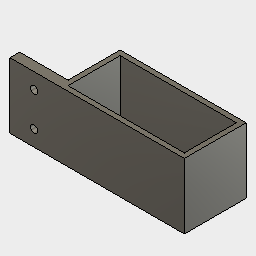
ServoHolder (Autodesk Fusion 360 design; units mm, degrees)
Autodesk Fusion 360 part; units mm, degrees
note: some values were not read from the file. Chosen so that the rebuilt part matches the saved one: which face or edge a step refers to.
sketch "Sketch1" plane through (0, 0, 0) normal (0, 1, 0) x (1, 0, 0)
  line L0 (0, 0) -> (47, 0) construction
  line L1 (47, 0) -> (47, 20.5) construction
  line L2 (47, 20.5) -> (0, 20.5) construction
  line L3 (0, 20.5) -> (0, 0) construction
  line L4 (-0.5, -0.5) -> (47.5, -0.5)
  line L5 (47.5, -0.5) -> (47.5, 21)
  line L6 (47.5, 21) -> (-0.5, 21)
  line L7 (-0.5, 21) -> (-0.5, -0.5)
  dimension "d1" = 47
  dimension "d2" = 20.5
  dimension "d3" = 0.5
  measures "d1" distance of L0.start L0.end
  measures "d2" distance of L0.start L2.end
extrude "Extrude1" add sketch "Sketch1" along normal blind 25 makes body 1
copy_body "Body->Comp1" bodies 1 removing the originals makes body 2 in component "ServoMount"
shell "Shell1" thickness 2 outward yes removed faces 0 bodies 2 in component "ServoMount"
extrude "Extrude1'" cut 1 faces at (14.8333, 27, -14.5) along direction (0, -1, 0) blind 2 on bodies 2 bodies 2 in component "ServoMount"
ref_plane "WorkPlane1" through (-2.5, 11.5, -10.25) normal (-1, 0, 0) x (0, 0, 1)
sketch "Sketch2" plane through (-2.5, 11.5, -10.25) normal (-1, 0, 0) x (0, 0, -1) in component "ServoMount"
  line L0 (-12.75, -13.5) -> (-8.75, -13.5)
  line L1 (-8.75, -13.5) -> (-8.75, 13.5)
  line L2 (-8.75, 13.5) -> (-12.75, 13.5)
  line L3 (-12.75, 13.5) -> (-12.75, -13.5)
  point P0 (-12.75, -13.5)
  dimension "d10" = 4
  measures "d10" distance of P0 L0.end
extrude "Extrude2" add sketch "Sketch2" along normal blind 20 bodies 2 in component "ServoMount"
ref_plane "WorkPlane2" through (-12.5, 11.5, -1.5) normal (0, 0, -1) x (0, -1, 0) in component "ServoMount"
sketch "Sketch3" plane through (-12.5, 11.5, -1.5) normal (0, 0, -1) x (1, 0, 0) in component "ServoMount"
  circle A0 centre (0, -7) radius 1.5
  line L0 (10, -13.5) -> (-10, -13.5)
  line L1 (-10, -13.5) -> (-10, 13.5)
  circle A1 centre (0, 7) radius 1.5
  line L2 (10, 13.5) -> (-10, 13.5)
  circle A2 centre (0, -7) radius 2.5
  circle A3 centre (0, 7) radius 2.5
  dimension "d14" = 3
  dimension "d15" = 6.5
  dimension "d16" = 10
  dimension "d17" = 3
  dimension "d18" = 10
  dimension "d19" = 6.5
  dimension "d24" = 1
  dimension "d25" = 1
  measures "d14" diameter of A0
  measures "d15" distance of A0.centre L0
  measures "d16" distance of A0.centre L1
  measures "d17" diameter of A1
  measures "d18" distance of L1 A1.centre
  measures "d19" distance of A1.centre L2
extrude "Extrude3" cut sketch "Sketch3" against normal up to surface (4 mm away) contours A0 bodies 2 in component "ServoMount"
extrude "Extrude4" cut sketch "Sketch3" against normal up to surface (4 mm away) contours A1 bodies 2 in component "ServoMount"
extrude "Extrude5" cut sketch "Sketch3" against normal blind 1 contours A2 bodies 2 in component "ServoMount"
extrude "Extrude6" cut sketch "Sketch3" against normal blind 1 contours A3 bodies 2 in component "ServoMount"
component "ServoMount" placed x (1, 0, 0) y (0, 1, 0) z (0, 0, 1) at (0, 0, 0)
